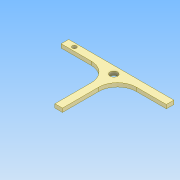
# Autodesk Inventor part: Top_Separator Lever
Saved by Autodesk Inventor 2018.1 (Build 221171000, 171)
## iProperties
Created: 2019-02-14
Part Number: Top_Separator Lever
Material: Nylon 6/6
Document SubType Name: Modeling
Designer: James
Density: 1.13 g/cm^3
Appearance: Nylon 6
Mass: 1.8781 g
Surface Area: 17.1526 cm^2
Volume: 1.66203 cm^3
Author: James
Autodesk Inventor part; units mm, degrees
ref_plane "YZ Plane" through (0, 0, 0) normal (1, 0, 0) x (0, 1, 0)
ref_plane "XZ Plane" through (0, 0, 0) normal (0, 1, 0) x (-1, 0, 0)
ref_plane "XY Plane" through (0, 0, 0) normal (0, 0, 1) x (1, 0, 0)
sketch "Sketch1" plane through (0, 0, 0) normal (0, 0, 1) x (1, 0, 0)
  line L0 (-39, 50) -> (6, 50)
  line L1 (6, 50) -> (6, 44)
  line L2 (6, 44) -> (-39, 44)
  line L3 (-39, 44) -> (-39, 50)
  line L4 (0, 44) -> (6, 44)
  line L5 (6, 44) -> (6, 0)
  line L6 (6, 0) -> (0, 0)
  line L7 (0, 0) -> (0, 44)
  line L8 (6, 50) -> (45, 50)
  line L9 (45, 50) -> (45, 44)
  line L10 (45, 44) -> (6, 44)
  line L11 (6, 44) -> (6, 50)
  dimension "d1" = 6
  dimension "d2" = 45
  dimension "d3" = 6
  dimension "d17" = 50
  dimension "d19" = 45
  constraints: 24 end point, 6 parallel, 3 coincident, 3 horizontal, 3 perpendicular, 1 point on line
  measures "d1" distance of L0.end L1.end
  measures "d2" distance of L0.start L0.end
  measures "d3" distance of L5.end L6.end
  measures "d17" distance between parallel lines of L6 L0
  measures "d19" distance between parallel lines of L7 L9
extrude "Extrusion1" add sketch "Sketch1" along normal blind 3
fillet "Fillet1" radius 15 2 edges at (0, 44, 1.5) (6, 44, 1.5)
sketch "Sketch2" plane through (0, 0, 3) normal (0, 0, 1) x (1, 0, 0)
  line L0 (45, 50) -> (-39, 50) projected
  line L1 (6, 0) -> (6, 29) projected
  point P0 (0, 0)
  point P1 (3, 44)
  point P2 (6, 44)
  dimension "d8" = 6
  dimension "d20" = 3
  measures "d8" distance from line of point (3, 44) L0
  measures "d20" distance from line of L1 point (3, 44)
hole "Hole1" at (3, 44, 3) direction (0, 0, -1) diameter 6 end through all
sketch "Sketch3" plane through (0, 0, 3) normal (0, 0, 1) x (1, 0, 0)
  line L0 (-39, 50) -> (-39, 44) projected
  point P0 (0, 0)
  point P1 (-31.5, 47)
  point P2 (-39, 47)
  dimension "d21" = 7.5
  constraints: 1 horizontal alignment, 1 midpoint
  measures "d21" distance from line of L0 point (-31.5, 47)
hole "Hole2" at (-31.5, 47, 3) direction (0, 0, -1) diameter 3.4 end through all clearance for "Flat Head Machine Screw" size "M3" standard "Ansi Metric M Profile"
equation "\"d19\" = d2"
body "Solid1"
